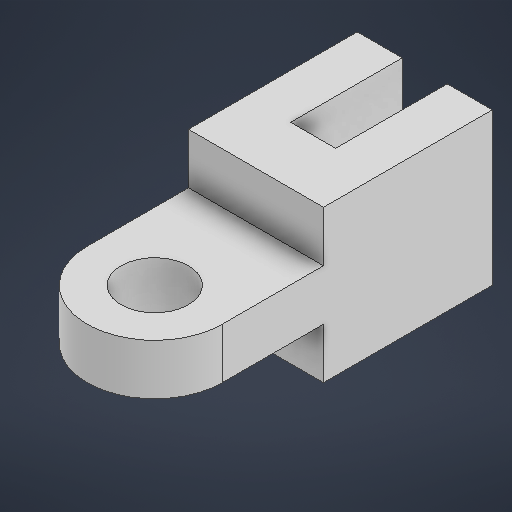
# Autodesk Inventor part: Part4
Saved by Autodesk Inventor 2026 (Build 300175050, 175E)
## iProperties
Created: 2026-03-19
Part Number: Part4
Material: Generic
Document SubType Name: Modeling
Designer: Administrator
Density: 1 g/cm^3
Appearance: Default
Author: Administrator
Autodesk Inventor part; units mm, degrees
ref_plane "YZ Plane" through (0, 0, 0) normal (1, 0, 0) x (0, 1, 0)
ref_plane "XZ Plane" through (0, 0, 0) normal (0, 1, 0) x (-1, 0, 0)
ref_plane "XY Plane" through (0, 0, 0) normal (0, 0, 1) x (1, 0, 0)
sketch "Sketch1" plane through (0, 0, 0) normal (1, 0, 0) x (0, 1, 0)
  line L0 (0, 0) -> (0, -30)
  line L1 (0, -30) -> (27, -30)
  line L2 (27, -30) -> (27, 0)
  line L3 (27, 0) -> (18, 0)
  line L4 (18, 0) -> (18, 30)
  line L5 (18, 30) -> (9, 30)
  line L6 (9, 30) -> (9, 0)
  line L7 (9, 0) -> (0, 0)
  dimension "d0" = 30
  dimension "d1" = 27
  dimension "d3" = 9
  dimension "d4" = 9
  dimension "d5" = 30
  constraints: 16 end point, 7 perpendicular, 1 point on line, 1 vertical
  measures "d0" distance of L0.start L0.end
  measures "d1" distance of L0.end L1.end
  measures "d3" distance of L6.end L0.start
  measures "d4" distance of L4.end L5.end
  measures "d5" distance of L3.end L4.end
extrude "Extrusion1" add sketch "Sketch1" along normal mid plane 24
fillet "Fillet1" radius 12 1 edges at (12, 13.5, 30)
fillet "Fillet2" radius 12 1 edges at (-12, 13.5, 30)
sketch "Sketch2" plane through (-12, 18, 0) normal (0, 1, 0) x (1, 0, 0)
  circle A0 centre (12, -18) radius 6
  line L0 (0, 0) -> (24, 0) projected
  line L1 (0, 30) -> (24, 30) projected
  point P0 (12, 0)
  dimension "d10" = 12
  dimension "d11" = 18
  constraints: 1 centre point
  measures "d10" diameter of A0
  measures "d11" distance from line of L0 A0.centre
sketch "Sketch3" plane through (-12, 27, 0) normal (0, 1, 0) x (1, 0, 0)
  line L0 (0, 30) -> (24, 30) projected
  line L1 (8, 30) -> (8, 10.1515)
  line L2 (8, 10.1515) -> (16, 10.1515)
  line L3 (16, 10.1515) -> (16, 30)
  line L4 (24, 30) -> (24, 0) projected
  line L5 (8, 30) -> (16, 30)
  point P0 (12, 0)
  dimension "d12" = 8
  dimension "d13" = 8
  constraints: 8 end point, 2 perpendicular, 2 point on line, 1 collinear, 1 vertical
  measures "d12" distance between parallel lines of L4 L3
  measures "d13" distance of L1.end L2.end
extrude "Extrusion2" cut sketch "Sketch2" against normal through all
extrude "Extrusion3" cut sketch "Sketch3" against normal through all
body "Solid1"
